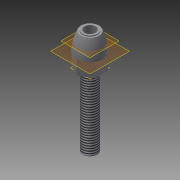
# Autodesk Inventor part: Adjustment screw
Saved by Autodesk Inventor 2014 SP2 (Build 180246200, 246)
## iProperties
Created: 2014-08-06
Part Number: Adjustment screw
Material: Generic
Document SubType Name: Modeling
Designer: Lukasz Szmit
Density: 1 g/cm^3
Appearance: Default
Author: Lukasz Szmit
Autodesk Inventor part; units mm, degrees
ref_plane "YZ Plane" through (0, 0, 0) normal (1, 0, 0) x (0, 1, 0)
ref_plane "XZ Plane" through (0, 0, 0) normal (0, 1, 0) x (-1, 0, 0)
sketch "Sketch2" plane through (0, 0, 0) normal (0, 0, 1) x (1, 0, 0)
  circle A0 centre (0, 0) radius 5
  dimension "d1" = 10
  constraints: 1 centre point, 1 coincident
  measures "d1" diameter of A0
sketch "Sketch3" plane through (0, 0, 0) normal (0, 0, 1) x (1, 0, 0)
  circle A0 centre (0, 0) radius 3.1
  dimension "d2" = 6.2
  constraints: 1 centre point, 1 coincident
  measures "d2" diameter of A0
sketch "Sketch4" plane through (0, 0, 0) normal (0, 0, 1) x (1, 0, 0)
  circle A0 centre (0, 0) radius 4.15
  dimension "d3" = 8.3
  constraints: 1 centre point, 1 coincident
  measures "d3" diameter of A0
ref_plane "Work Plane5" through (0, 0, -10) normal (0, 0, 1) x (1, 0, 0)
sketch "Sketch5" plane through (0, 0, -10) normal (0, 0, 1) x (1, 0, 0)
  circle A0 centre (0, 0) radius 7.5055
  dimension "d9" = 15.011
  constraints: 1 centre point
  measures "d9" diameter of A0
ref_plane "Work Plane3" through (0, 0, -5) normal (0, 0, 1) x (1, 0, 0)
sketch "Sketch6" plane through (0, 0, -5) normal (0, 0, 1) x (1, 0, 0)
  circle A0 centre (0, 0) radius 6.75
  dimension "d11" = 13.5
  constraints: 1 centre point, 1 coincident
  measures "d11" diameter of A0
loft "Loft1" add profiles "Sketch5", "Sketch6", "Sketch2"
extrude "Extrusion2" add sketch "Sketch4" along normal blind 0.5
extrude "Extrusion3" cut sketch "Sketch3" along normal blind 0.5 and the other way blind 10
ref_plane "Work Plane4" through (0, 0, -18) normal (0, 0, 1) x (1, 0, 0)
sketch "Sketch8" plane through (0, 0, -18) normal (0, 0, 1) x (1, 0, 0)
  line L0 (0, 7.5056) -> (6.5, 3.7528)
  line L1 (6.5, 3.7528) -> (6.5, -3.7528)
  line L2 (6.5, -3.7528) -> (0, -7.5056)
  line L3 (0, -7.5056) -> (-6.5, -3.7528)
  line L4 (-6.5, -3.7528) -> (-6.5, 3.7528)
  line L5 (-6.5, 3.7528) -> (0, 7.5056)
  point P0 (0, 0)
  point P1 (0, 0)
  dimension "d27" = 13
  constraints: 12 end point, 1 coincident, 13 other
  measures "d27" distance between parallel lines of L4 L1
extrude "Extrusion4" add sketch "Sketch8" along normal blind 8
sketch "Sketch9" plane through (0, 0, -18) normal (0, 0, -1) x (-1, 0, 0)
  circle A0 centre (0, 0) radius 4
  dimension "d30" = 8
  constraints: 1 centre point, 1 coincident
  measures "d30" diameter of A0
extrude "Extrusion5" add sketch "Sketch9" along normal blind 40
sketch "Sketch10" plane through (0, 0, -58) normal (0, 0, -1) x (-1, 0, 0)
  circle A0 centre (0, 0) radius 4 projected
  circle A1 centre (0, 0) radius 1
  dimension "d33" = 2
  constraints: 1 centre point, 1 coincident
  measures "d33" diameter of A1
extrude "Extrusion6" cut sketch "Sketch10" against normal blind 40 contours A1
sketch "Sketch11" plane through (0, 0, -18) normal (0, 0, -1) x (-1, 0, 0)
  circle A0 centre (0, 0) radius 4 projected
  circle A1 centre (0, 0) radius 1
  dimension "d36" = 2
  constraints: 1 centre point, 1 coincident
  measures "d36" diameter of A1
extrude "Extrusion7" cut sketch "Sketch11" against normal blind 8 contours A1
thread "Thread1" size "M8x1.25" class "6g" standard "ISO Metric profile" length 38
fillet "Fillet1" radius 1.5 1 edges at (4, 0, -18)
body "Solid2"
